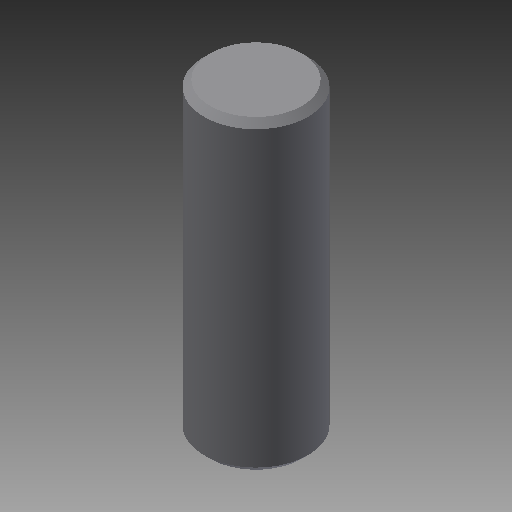
# Autodesk Inventor part: FO-090.751.468NT-00_rod-bif
Saved by Autodesk Inventor 2019.4 (Build 234330000, 330)
## iProperties
Category: PARTsolutions
Company: BIMBA
Created: 2020-02-04
Part Number: FO-090.751.468NT-00_rod-bif
Material: Generic
Catalog Web Link: www.cadenas.de
Description: FO1 Basic Model Rod-Bimba FLAT-1
Vendor: BIMBA
Document SubType Name: Modeling
Designer: psadmin
Manufacturer: BIMBA
Mass: 4.70119 g
Surface Area: 17.0392 cm^2
Volume: 4.70119 cm^3
Density: 1 g/cm^3
Appearance: PSOLRGB-180-180-180
PSOL_IDENT_0: {$CADENAS_DATA\23d-libs\bimba\bimba_brand\bimba_imperial\bimba_full_line\flat_cylinders\fo1\fo1_basi
PSOL_IDENT_1: c_model_rod.prj},304 {VTYP=3D},{NB=FO-090.751.468NT-00_rod-bif},{LINA=FO-090.751.468NT-00_rod-bif},{
PSOL_IDENT_2: NN=FO1 Basic Model Rod},{DATE=22.01.2020 09:06:03},{GEOMDATE=12.12.2018 07:59:21},{VERSION=},{LINEID=
PSOL_IDENT_3: 30},{WBVAR=STROKE,ACTING,MNTR,MNTF,HR,FS,LENGTH,STPT1,STPT2,STPT3,RT,M,W,UM,MRS,FCD,RCD},{WBNUMERIC=
PSOL_IDENT_4: STROKE,LENGTH,FCD,RCD}  {NB=FO-090.751.468NT-00_rod-bif},{LINA=FO-090.751.468NT-00_rod-bif},{KT=DUMM
PSOL_IDENT_5: Y},{PN=FO-090.751.468NT-00},{PN2=FO-090.751.468NT-00},{BORE=1.06250000},{BOREPN=09},{BORE1=1.062},{S
PSOL_IDENT_6: TROKE=0.75000},{STROKEMIN=0.735},{STROKEMAX=16},{ACTING=},{ACTINGALG='','Double Acting, Single End R
PSOL_IDENT_7: od [FO]', 'D'  , 'Double Acting, Double End Rod [FOD]', 'R', 'Reverse Acting [FOR]', 'S'  ,'Single A
PSOL_IDENT_8: cting [FOS]'},{MNTR=},{MNTF=},{MNTFALG='','Standard Counterbored Mounting Holes','2F','Trunnion Moun
PSOL_IDENT_9: t, Front','3F','Threaded Mounting Holes, Front','4F','Screw Clearance Holes, Front','5','Nose Mount'
PSOL_IDENT_10: },{HR=},{HRALG='','N/A'},{FS=},{LENGTHALG=[0.735:100/0.001]},{LENGTH=1.46800},{STPT1=},{STPT1ALG= ''
PSOL_IDENT_11: , 'N/A' },{STPT2=},{STPT2ALG= '' , 'N/A' },{STPT3=},{STPT3ALG= '' , 'N/A' },{RT=NT},{M=},{W=},{UM=}
PSOL_IDENT_12: ,{MRS=},{MRSALG='','None ','Z','Metallic Rod Scraper [Z]'},{MALG='','Without Magnetic Position Sensi
PSOL_IDENT_13: ng','M','With Magnetic Position Sensing [M]','M1','With Magnetic Position Sensing 1 [M1]','M3','With
PSOL_IDENT_14: Magnetic Position Sensing 3 [M3]' },{EE=},{EEALG='','Without Extra Extension','EE','With Extra Exte
PSOL_IDENT_15: nsion'},{EELALG=0},{EELMAX=19.25},{EEL=0},{EELPN=},{A=2.00000000},{BA=0.88000},{BB=0.94000},{BC=0.88
PSOL_IDENT_16: },{BD=1.38},{C=1.69000000},{DD=4.00000000},{D=0.13800000},{CPIL=0.15600000},{DC=0.25000000},{DCP=0.1
PSOL_IDENT_17: 4800000},{DCD=1.68700000},{ES=0.31250000},{EC=0.31250000},{ED=0.70000000},{F=0.50000000},{H=0.435500
PSOL_IDENT_18: 00},{J=0.50000000},{J2=0.500},{K=0.25000000},{L=0.40500000},{LDP=0.32300000},{LP=0.12500000},{LPDP=0
PSOL_IDENT_19: .59000000},{TD=1.11200000},{TDDP=0.21800},{TD1=1.10900},{TD2=1.12200},{TDIN=1.06200},{LSF=0.00000000
PSOL_IDENT_20: },{LSFDP=0.00000000},{BC1=0.88000},{BC2=1.50000},{BC3=2.13000},{BC4=2.75000},{BD1=1.38000},{BD2=2.00
PSOL_IDENT_21: 000},{BD3=2.63000},{BD4=3.25000},{MT=0.31250000},{CMT=0.31250000},{LG=0.50000000},{HF=0.22000000},{H
PSOL_IDENT_22: M=0.16000000},{HD=},{HALG=0},{HDY=0},{HDH=1.468},{LG1=0.00000000},{FCD=0},{RCD=0},{NPT=0.405},{FTL1=
PSOL_IDENT_23: 0.700},{FTLSR=0.325},{TDD=0.825},{TDDSR=0.450},{TDDSRC=0.492},{TDDC=0.867},{NPTTDD=0.421},{FTL=0.700
PSOL_IDENT_24: },{TDDR=0.825},{TDDRC=0.867},{WD=0.480},{TL=0.135},{HRID=0.218},{HRNTP=0.159},{HRMT=0.159},{GL=0.066
PSOL_IDENT_25: },{GD=0.247},{GR=0.034},{GLC=0.086},{GDC=0.229},{GRC=0.034},{NR=1.000},{RTALG='', 'Standard', 'CFT',
PSOL_IDENT_26: 'Coarse Female Thread', 'CMT'  , 'Male Rod Thread (Coarse)','MT', 'Male Rod End (Fine)', 'NT'  , 'N
PSOL_IDENT_27: on-Threaded Rod'},{RDEEP=0},{LDEEP=0.825},{DEEP2=0.825},{RL=1.973},{BBB=0.88},{RL22=0.125},{FSADD=0}
PSOL_IDENT_28: ,{HDADD=0},{MADD=0},{AC2=0},{MADD1=0.88},{HDADD1=0.190},{FSADD1=0.380},{UMALG='','Without Magnetic P
PSOL_IDENT_29: osition Sensing 90','U','With Magnetic Position Sensing 90 [U]','U1','With Magnetic Position Sensing
PSOL_IDENT_30: 90 Position 1 [U1]','U3','With Magnetic Position Sensing 90 Position 3 [U3]' },{FSALG='','Standard
PSOL_IDENT_31: Friction Seals','L','Low Friction Seals', 'X', 'Ring Rod Seal'},{MNTRALG='','Standard Counterbored M
PSOL_IDENT_32: ounting Holes','1','Pivot Mount','1N','Pivot Mount 90 Deg. from Standard','2R','Trunnion Mount, Rear'
PSOL_IDENT_33: ,'3R','Threaded Mounting Holes, Rear','4R','Screw Clearance Holes, Rear'},{AC1=0.750},{WALG='', 'Wit
PSOL_IDENT_34: hout Wiper', 'W', 'With Wiper'},{M1=0.880},{M2=0.880},{M3=0.880},{MNT4F=,'4F','Screw Clearance Holes
PSOL_IDENT_35: , Front'},{FTLF=0.700},{FTLR=0.7}
NN: FO1 Basic Model Rod
NT: Bimba FLAT-1
NB: FO-090.751.468NT-00_rod-bif
NBSYN: $PN2._rod-bif
LINA: FO-090.751.468NT-00_rod-bif
PN: FO-090.751.468NT-00
BORE: 0
BOREPN: 09
BORE1: 1.062
STROKE: 0.75
ACTING: Double Acting, Single End Rod [FO]
MNTR: Standard Counterbored Mounting Holes
MNTF: Standard Counterbored Mounting Holes
HR: N/A
FS: Standard Friction Seals
LENGTH: 1.468
STPT1: N/A
STPT2: N/A
STPT3: N/A
RT: Non-Threaded Rod
M: Without Magnetic Position Sensing
W: Without Wiper
UM: Without Magnetic Position Sensing 90
A: 2
BA: 0.88
BB: 0.94
C: 1.69
DD: 4
D: 0.138
CPIL: 0.156
DC: 0.25
DCP: 0.148
DCD: 1.687
ES: 0.3125
EC: 0.3125
ED: 0.7
F: 0.5
H: 0.4355
J: 0.5
J2: 0.5
K: 0.25
L: 0.405
LDP: 0.323
LP: 0.125
LPDP: 0.59
TD: 1.112
TDDP: 0.218
TD1: 1.109
TD2: 1.122
TDIN: 1.062
LSF: 0
LSFDP: 0
BC1: 0.88
BC2: 1.5
BC3: 2.13
BC4: 2.75
BD1: 1.38
BD2: 2
BD3: 2.63
BD4: 3.25
MT: 0.3125
CMT: 0.3125
LG: 0.5
HF: 0.22
HM: 0.16
FCD: 0
RCD: 0
NPT: 0.405
FTL1: 0.7
FTLSR: 0.325
TDD: 0.825
TDDSR: 0.45
TDDSRC: 0.492
TDDC: 0.867
NPTTDD: 0.421
WD: 0.48
TL: 0.135
HRID: 0.218
HRNTP: 0.159
HRMT: 0.159
GL: 0.066
GD: 0.247
GR: 0.034
GLC: 0.086
GDC: 0.229
GRC: 0.034
NR: 1
HDADD1: 0.19
FSADD1: 0.38
AC1: 0.75
M1: 0.88
M2: 0.88
M3: 0.88
SUPPLIER: BIMBA
ARTICLENO: FO-090.751.468NT-00_rod-bif
BOMINFO: FO-090.751.468NT-00_rod-bif
CREATOR: CADENAS GmbH
Title: FO-090.751.468NT-00_rod-bif
Author: Cadenas PARTsolutions
Comments: Bimba FLAT-1
Autodesk Inventor part; units mm, degrees
sketch "Sketch_10" plane through (0, 0, 0) normal (0, 0, 1) x (1, 0, 0)
  line L0 (0, 0) -> (0, 37.2872)
  line L1 (0, 37.2872) -> (5.588, 37.2872)
  line L2 (5.588, 37.2872) -> (6.35, 36.5252)
  line L3 (6.35, 36.5252) -> (6.35, 0.762)
  line L4 (6.35, 0.762) -> (5.588, 0)
  line L5 (5.588, 0) -> (0, 0)
  line L6 (0, 0) -> (0, 37.2872)
  constraints: 14 end point
revolve "Revolution1" add sketch "Sketch_10" angle 360 about axis through (0, 0, 0) along (0, -1, 0)
ref_plane "b11_XY" through (0, 0, 0) normal (0, 1, 0) x (1, 0, 0)
ref_plane "b11_YZ" through (0, 0, 0) normal (1, 0, 0) x (0, 0, -1)
ref_plane "b11_ZX" through (0, 0, 0) normal (0, 0, -1) x (0, 1, 0)
ref_plane "b2_XY" through (0, 37.2872, 0) normal (0, 1, 0) x (1, 0, 0)
ref_plane "b2_YZ" through (0, 37.2872, 0) normal (1, 0, 0) x (0, 0, -1)
ref_plane "b2_ZX" through (0, 37.2872, 0) normal (0, 0, -1) x (0, 1, 0)
ref_plane "f1_XY" through (0, 37.2872, 6.35) normal (1, 0, 0) x (0, 0, -1)
ref_plane "f1_YZ" through (0, 37.2872, 6.35) normal (0, 0, -1) x (0, 1, 0)
ref_plane "f1_ZX" through (0, 37.2872, 6.35) normal (0, 1, 0) x (1, 0, 0)
ref_plane "f2_XY" through (0, 37.2872, -6.35) normal (1, 0, 0) x (0, 0, -1)
ref_plane "f2_YZ" through (0, 37.2872, -6.35) normal (0, 0, -1) x (0, 1, 0)
ref_plane "f2_ZX" through (0, 37.2872, -6.35) normal (0, 1, 0) x (1, 0, 0)
ref_plane "h1_XY" through (-5.5309, 37.2872, 0) normal (0, 1, 0) x (1, 0, 0)
ref_plane "h1_YZ" through (-5.5309, 37.2872, 0) normal (1, 0, 0) x (0, 0, -1)
ref_plane "h1_ZX" through (-5.5309, 37.2872, 0) normal (0, 0, -1) x (0, 1, 0)
ref_plane "h2_XY" through (5.5309, 37.2872, 0) normal (0, 1, 0) x (1, 0, 0)
ref_plane "h2_YZ" through (5.5309, 37.2872, 0) normal (1, 0, 0) x (0, 0, -1)
ref_plane "h2_ZX" through (5.5309, 37.2872, 0) normal (0, 0, -1) x (0, 1, 0)
ref_plane "npt1_XY" through (0, 37.2872, 5.1435) normal (0, 1, 0) x (1, 0, 0)
ref_plane "npt1_YZ" through (0, 37.2872, 5.1435) normal (1, 0, 0) x (0, 0, -1)
ref_plane "npt1_ZX" through (0, 37.2872, 5.1435) normal (0, 0, -1) x (0, 1, 0)
ref_plane "npt1_1_XY" through (0, 0, 5.1435) normal (0, 1, 0) x (1, 0, 0)
ref_plane "npt1_1_YZ" through (0, 0, 5.1435) normal (1, 0, 0) x (0, 0, -1)
ref_plane "npt1_1_ZX" through (0, 0, 5.1435) normal (0, 0, -1) x (0, 1, 0)
ref_plane "npt2_XY" through (0, 37.2872, -5.1435) normal (0, 1, 0) x (1, 0, 0)
ref_plane "npt2_YZ" through (0, 37.2872, -5.1435) normal (1, 0, 0) x (0, 0, -1)
ref_plane "npt2_ZX" through (0, 37.2872, -5.1435) normal (0, 0, -1) x (0, 1, 0)
ref_plane "npt2_1_XY" through (0, 0, -5.1435) normal (0, 1, 0) x (1, 0, 0)
ref_plane "npt2_1_YZ" through (0, 0, -5.1435) normal (1, 0, 0) x (0, 0, -1)
ref_plane "npt2_1_ZX" through (0, 0, -5.1435) normal (0, 0, -1) x (0, 1, 0)
ref_plane "rod_XY" through (0, 0, 0) normal (0, 1, 0) x (1, 0, 0)
ref_plane "rod_YZ" through (0, 0, 0) normal (1, 0, 0) x (0, 0, -1)
ref_plane "rod_ZX" through (0, 0, 0) normal (0, 0, -1) x (0, 1, 0)
ref_plane "rod_to_part_XY" through (0, 0, 0) normal (0, 1, 0) x (1, 0, 0)
ref_plane "rod_to_part_YZ" through (0, 0, 0) normal (1, 0, 0) x (0, 0, -1)
ref_plane "rod_to_part_ZX" through (0, 0, 0) normal (0, 0, -1) x (0, 1, 0)
ref_plane "th1_XY" through (0, 37.2872, 3.9688) normal (0, 1, 0) x (1, 0, 0)
ref_plane "th1_YZ" through (0, 37.2872, 3.9688) normal (1, 0, 0) x (0, 0, -1)
ref_plane "th1_ZX" through (0, 37.2872, 3.9688) normal (0, 0, -1) x (0, 1, 0)
ref_plane "th2_XY" through (0, 37.2872, -3.9688) normal (0, 1, 0) x (1, 0, 0)
ref_plane "th2_YZ" through (0, 37.2872, -3.9688) normal (1, 0, 0) x (0, 0, -1)
ref_plane "th2_ZX" through (0, 37.2872, -3.9688) normal (0, 0, -1) x (0, 1, 0)
ref_plane "to_rod_pivot_XY" through (0, 37.2872, 0) normal (0, 1, 0) x (1, 0, 0)
ref_plane "to_rod_pivot_YZ" through (0, 37.2872, 0) normal (1, 0, 0) x (0, 0, -1)
ref_plane "to_rod_pivot_ZX" through (0, 37.2872, 0) normal (0, 0, -1) x (0, 1, 0)
ref_plane "to_rod_pivot1_XY" through (0, 0, 0) normal (0, 1, 0) x (1, 0, 0)
ref_plane "to_rod_pivot1_YZ" through (0, 0, 0) normal (1, 0, 0) x (0, 0, -1)
ref_plane "to_rod_pivot1_ZX" through (0, 0, 0) normal (0, 0, -1) x (0, 1, 0)
body "Solid1"
